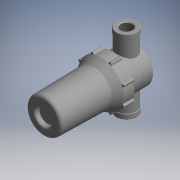
# Autodesk Inventor part: 547261 VAF-DB-1/4
Saved by Autodesk Inventor 2017.3 (Build 213256000, 256)
## iProperties
Part Number: 547261 VAF-DB-1/4
Material: Generic
Catalog Web Link: www.cadenas.de
Description: VAF-Accessories for vacuum
Vendor: FESTO
Document SubType Name: Modeling
Designer: partserver
Manufacturer: FESTO
Mass: 71 g
Surface Area: 182.991 cm^2
Volume: 114.297 cm^3
Density: 1 g/cm^3
Appearance: PSOLRGB-175-175-175
Category: PARTsolutions
Company: FESTO
Title: 547261 VAF-DB-1/4
Author: Cadenas PARTsolutions
Comments: Accessories for vacuum
PSOL_IDENT_0: {$CADENAS_DATA\23d-libs\festo\parts\v\vaf\vaf.prj},171 {VTYP=3D},{NB=547261 VAF-DB-1/4},{LINA=547261
PSOL_IDENT_1: VAF-DB-1/4},{NN=VAF},{DATE=24.04.2020 08:24:54},{GEOMDATE=08.04.2020 10:45:48},{VERSION=},{LINEID=4
PSOL_IDENT_2: 0},{WBVAR=},{WBNUMERIC=}  {NB=547261 VAF-DB-1/4},{LINA=547261 VAF-DB-1/4},{KT=DUMMY},{TNR=547261},{T
PSOL_IDENT_3: YP=VAF-DB-1/4},{WGT=71.000},{VER=3},{VER2=1.000},{D1=0},{D2=0},{D3=0.00},{L=0.0},{SW=0},{A=75.0},{B=
PSOL_IDENT_4: 94.5},{C=84.5},{G=1/4},{GA=13.157},{L1=0},{L2=0},{L3=0},{L4=0},{L5=0},{L6=0},{L7=0.0},{L8=0.0},{UR=1
PSOL_IDENT_5: 5.000},{L9=0.000},{CNSMASSEXACT=0.071}
NB: 547261 VAF-DB-1/4
NN: VAF
NT: Accessories for vacuum
NBSYN: $TNR. $TYP.
LINA: 547261 VAF-DB-1/4
CATALOG: Festo
TNR: 547261
TYP: VAF-DB-1/4
D1: 0
D2: 0
D3: 0
L: 0
SW: 0
A: 75
B: 94.5
C: 84.5
G: 1/4
L1: 0
L2: 0
L3: 0
L4: 0
L5: 0
L6: 0
L7: 0
L8: 0
L9: 0
CNSMASSEXACT: 0.071
SUPPLIER: FESTO
ARTICLENO: 547261 VAF-DB-1/4
BOMINFO: 547261 VAF-DB-1/4
CREATOR: CADENAS GmbH
Autodesk Inventor part; units mm, degrees
ref_plane "YZ Plane" through (0, 0, 0) normal (1, 0, 0) x (0, 1, 0)
ref_plane "XZ Plane" through (0, 0, 0) normal (0, 1, 0) x (-1, 0, 0)
ref_plane "XY Plane" through (0, 0, 0) normal (0, 0, 1) x (1, 0, 0)
sketch "Sketch_8" plane through (0, 0, 0) normal (1, 0, 0) x (0, 1, 0)
  line L0 (-15, 0) -> (10, 0)
  line L1 (10, 0) -> (10, -18)
  line L2 (10, -18) -> (-15, -18)
  line L3 (-15, -18) -> (-15, 0)
  line L4 (-15, 0) -> (10, 0)
  constraints: 10 end point
revolve "Revolution1" add sketch "Sketch_8" angle 360 about axis through (0, -15, 0) along (0, -1, 0)
sketch "Sketch_9" plane through (0, 0, 0) normal (1, 0, 0) x (0, 1, 0)
  circle A0 centre (0, 0) radius 7.5
  constraints: 1 centre point
extrude "Extrusion1" cut sketch "Sketch_9" along normal mid plane 100
sketch "Sketch_2" plane through (0, 0, 0) normal (1, 0, 0) x (0, 1, 0)
  line L0 (-15, 0) -> (10, 0)
  line L1 (10, 0) -> (10, -17.9)
  line L2 (10, -17.9) -> (-15, -17.9)
  line L3 (-15, -17.9) -> (-15, 0)
  line L4 (-15, 0) -> (10, 0)
  constraints: 10 end point
revolve "Revolution2" add sketch "Sketch_2" angle 360 about axis through (0, -15, 0) along (0, -1, 0)
sketch "Sketch_11" plane through (0, 0, 0) normal (1, 0, 0) x (0, 1, 0)
  line L0 (-0.75, 6) -> (-0.75, -3)
  line L1 (-0.75, -3) -> (-1.7321, -3)
  line L2 (-1.7321, -3) -> (0, -6)
  line L3 (0, -6) -> (1.7321, -3)
  line L4 (1.7321, -3) -> (0.75, -3)
  line L5 (0.75, -3) -> (0.75, 6)
  line L6 (0.75, 6) -> (-0.75, 6)
  constraints: 14 end point
extrude "Extrusion2" add sketch "Sketch_11" along normal mid plane 60
sketch "Sketch_12" plane through (0, 0, 0) normal (1, 0, 0) x (0, 1, 0)
  line L0 (-15, 0) -> (10, 0)
  line L1 (15, -5) -> (10, -5)
  line L2 (10, -5) -> (10, -16.5)
  arc A0 (8.5, -18) -> (10, -16.5) centre (8.5, -16.5) ccw
  line L3 (8.5, -18) -> (-15, -18)
  line L4 (-15, -18) -> (-15, -5)
  line L5 (-15, -5) -> (-20, -5)
  line L6 (-20, -5) -> (-20, -100)
  line L7 (-20, -100) -> (15, -100)
  line L8 (15, -100) -> (15, -5)
  constraints: 18 end point, 2 point on circle, 1 centre point
revolve "Revolution3" cut sketch "Sketch_12" angle 360 about axis through (0, -15, 0) along (0, -1, 0)
sketch "Sketch_13" plane through (0, 0, 0) normal (1, 0, 0) x (0, 1, 0)
  line L0 (-80.14, 0) -> (-15, 0)
  line L1 (-15, 0) -> (-15, -23)
  line L2 (-15, -23) -> (-25.6915, -23)
  line L3 (-25.6915, -23) -> (-33.3612, -18.5719)
  line L4 (-33.3612, -18.5719) -> (-81.5524, -17.7307)
  arc A0 (-84.5, -14.7311) -> (-81.5524, -17.7307) centre (-81.5, -14.7312) ccw
  line L5 (-84.5, -14.7311) -> (-84.5, -10.6561)
  arc A1 (-82.8473, -8.6865) -> (-84.5, -10.6561) centre (-82.5, -10.6561) ccw
  line L6 (-82.8473, -8.6865) -> (-80.9664, -8.3548)
  arc A2 (-80.9664, -8.3548) -> (-80.14, -7.37) centre (-81.14, -7.37) ccw
  line L7 (-80.14, -7.37) -> (-80.14, 0)
  line L8 (-80.14, 0) -> (-15, 0)
  constraints: 18 end point, 6 point on circle, 3 centre point
revolve "Revolution4" add sketch "Sketch_13" angle 360 about axis through (0, -80.14, 0) along (0, -1, 0)
sketch "Sketch_14" plane through (0, 0, 0) normal (1, 0, 0) x (0, 1, 0)
  line L0 (0, -37.5) -> (0, 37.5)
  line L1 (0, 37.5) -> (9.9, 37.5)
  arc A0 (10.4, 37) -> (9.9, 37.5) centre (9.9, 37) ccw
  line L2 (10.4, 37) -> (10.4, 33)
  arc A1 (9.9, 32.5) -> (10.4, 33) centre (9.9, 33) ccw
  line L3 (9.9, 32.5) -> (9.9, -32.5)
  arc A2 (10.4, -33) -> (9.9, -32.5) centre (9.9, -33) ccw
  line L4 (10.4, -33) -> (10.4, -37)
  arc A3 (9.9, -37.5) -> (10.4, -37) centre (9.9, -37) ccw
  line L5 (9.9, -37.5) -> (0, -37.5)
  line L6 (0, -37.5) -> (0, 37.5)
  constraints: 14 end point, 8 point on circle, 4 centre point
revolve "Revolution5" add sketch "Sketch_14" angle 360 about axis through (0, 0, -37.5) along (0, 0, -1)
sketch "Sketch_3" plane through (0, 0, 0) normal (1, 0, 0) x (0, 1, 0)
  line L0 (0, 18.5) -> (0, 37.5)
  line L1 (0, 37.5) -> (6.5785, 37.5)
  line L2 (6.5785, 37.5) -> (5.7225, 36.644)
  line L3 (5.7225, 36.644) -> (5.7225, 18.5)
  line L4 (5.7225, 18.5) -> (0, 18.5)
  line L5 (0, 18.5) -> (0, 37.5)
  constraints: 12 end point
revolve "Revolution6" cut sketch "Sketch_3" angle 360 about axis through (0, 0, 18.5) along (0, 0, -1)
thread "Thread1" size "G13.157x1.337" designation "G 1/4" standard "ISO Pipe Threads" full length
sketch "Sketch_15" plane through (0, 0, 0) normal (1, 0, 0) x (0, 1, 0)
  line L0 (0, -37.5) -> (0, -18.5)
  line L1 (0, -18.5) -> (5.7225, -18.5)
  line L2 (5.7225, -18.5) -> (5.7225, -36.644)
  line L3 (5.7225, -36.644) -> (6.5785, -37.5)
  line L4 (6.5785, -37.5) -> (0, -37.5)
  line L5 (0, -37.5) -> (0, -18.5)
  constraints: 12 end point
revolve "Revolution7" cut sketch "Sketch_15" angle 360 about axis through (0, 0, -37.5) along (0, 0, -1)
thread "Thread2" size "G13.157x1.337" designation "G 1/4" standard "ISO Pipe Threads" full length
sketch "Sketch_4" plane through (0, -15, 0) normal (0, 1, 0) x (1, 0, 0)
  arc A0 (-22.3036, 10.1758) -> (-22.9665, 8.5756) centre (-22.1731, 9.1844) ccw
  line L0 (-22.9665, 8.5756) -> (-21.7902, 7.0427)
  arc A1 (-21.7902, 7.0427) -> (-21.7902, -7.0427) centre (0, 0) ccw
  line L1 (-21.7902, -7.0427) -> (-22.9665, -8.5756)
  arc A2 (-22.9665, -8.5756) -> (-22.3036, -10.1758) centre (-22.1731, -9.1844) ccw
  line L2 (-22.3036, -10.1758) -> (-20.3879, -10.4281)
  arc A3 (-20.3879, -10.4281) -> (-10.4281, -20.3879) centre (0, 0) ccw
  line L3 (-10.4281, -20.3879) -> (-10.1758, -22.3036)
  arc A4 (-10.1758, -22.3036) -> (-8.5756, -22.9665) centre (-9.1844, -22.1731) ccw
  line L4 (-8.5756, -22.9665) -> (-7.0427, -21.7902)
  arc A5 (-7.0427, -21.7902) -> (7.0427, -21.7902) centre (0, 0) ccw
  line L5 (7.0427, -21.7902) -> (8.5756, -22.9665)
  arc A6 (8.5756, -22.9665) -> (10.1758, -22.3036) centre (9.1844, -22.1731) ccw
  line L6 (10.1758, -22.3036) -> (10.4281, -20.3879)
  arc A7 (10.4281, -20.3879) -> (20.3879, -10.4281) centre (0, 0) ccw
  line L7 (20.3879, -10.4281) -> (22.3036, -10.1758)
  arc A8 (22.3036, -10.1758) -> (22.9665, -8.5756) centre (22.1731, -9.1844) ccw
  line L8 (22.9665, -8.5756) -> (21.7902, -7.0427)
  arc A9 (21.7902, -7.0427) -> (21.7902, 7.0427) centre (0, 0) ccw
  line L9 (21.7902, 7.0427) -> (22.9665, 8.5756)
  arc A10 (22.9665, 8.5756) -> (22.3036, 10.1758) centre (22.1731, 9.1844) ccw
  line L10 (22.3036, 10.1758) -> (20.3879, 10.4281)
  arc A11 (20.3879, 10.4281) -> (10.4281, 20.3879) centre (0, 0) ccw
  line L11 (10.4281, 20.3879) -> (10.1758, 22.3036)
  arc A12 (10.1758, 22.3036) -> (8.5756, 22.9665) centre (9.1844, 22.1731) ccw
  line L12 (8.5756, 22.9665) -> (7.0427, 21.7902)
  arc A13 (7.0427, 21.7902) -> (-7.0427, 21.7902) centre (0, 0) ccw
  line L13 (-7.0427, 21.7902) -> (-8.5756, 22.9665)
  arc A14 (-8.5756, 22.9665) -> (-10.1758, 22.3036) centre (-9.1844, 22.1731) ccw
  line L14 (-10.1758, 22.3036) -> (-10.4281, 20.3879)
  arc A15 (-10.4281, 20.3879) -> (-20.3879, 10.4281) centre (0, 0) ccw
  line L15 (-20.3879, 10.4281) -> (-22.3036, 10.1758)
  constraints: 32 end point, 32 point on circle, 16 centre point
extrude "Extrusion3" add sketch "Sketch_4" against normal blind 10.66
sketch "Sketch_23" plane through (0, 0, 0) normal (0, 0, 1) x (1, 0, 0)
  line L0 (11.335, 10) -> (11.335, 5)
  line L1 (11.335, 5) -> (10.335, 5)
  line L2 (10.335, 5) -> (9.8976, 10)
  line L3 (9.8976, 10) -> (11.335, 10)
  line L4 (11.335, 10) -> (11.335, 5)
  constraints: 10 end point
revolve "Revolution8" cut sketch "Sketch_23" angle 360 about axis through (11.335, 10, 0) along (0, -1, 0)
sketch "Sketch_24" plane through (0, 0, 0) normal (0, 0, 1) x (1, 0, 0)
  line L0 (-11.335, 10) -> (-11.335, 5)
  line L1 (-11.335, 5) -> (-12.335, 5)
  line L2 (-12.335, 5) -> (-12.7724, 10)
  line L3 (-12.7724, 10) -> (-11.335, 10)
  line L4 (-11.335, 10) -> (-11.335, 5)
  constraints: 10 end point
revolve "Revolution9" cut sketch "Sketch_24" angle 360 about axis through (-11.335, 10, 0) along (0, -1, 0)
body "Solid1"
